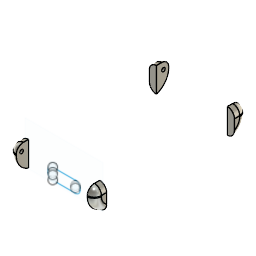
ILY Bracelet v2 v3 (Autodesk Fusion 360 design; units mm, degrees)
Autodesk Fusion 360 part; units mm, degrees
note: some values were not read from the file. Chosen so that the rebuilt part matches the saved one: which bodies a step acts on; which pieces of a blend or face edit are solid. Set by a fixed rule: which sketch regions a step uses.
sketch "Sketch1" plane through (0, 0, 0) normal (0, 0, 1) x (1, 0, 0)
  line L0 (0, 0) -> (22, 0)
  line L1 (22, 0) -> (22, 36)
  line L2 (22, 36) -> (0, 36)
  line L3 (0, 36) -> (0, 0)
  line L4 (1, 0.5) -> (21, 0.5)
  line L5 (21, 0.5) -> (21, 35)
  line L6 (21, 35) -> (1, 35)
  line L7 (1, 35) -> (1, 0.5)
  spline S0 degree 3 poles (15.3516, 13.4274) (15.5498, 13.4655) (15.7406, 13.3283) (15.7771, 13.115) knots 0 0 0 0 1 1 1 1
  spline S1 degree 3 poles (4.4385, 20.9712) (5.1653, 22.038) (6.0895, 22.8762) (7.1909, 23.4629) knots 0 0 0 0 1 1 1 1
  spline S2 degree 3 poles (10.9559, 18.0921) (10.1119, 18.0921) (9.4293, 17.4292) (9.4293, 16.6138) knots 0 0 0 0 1 1 1 1
  arc A0 (15.3516, 13.4274) -> (14.5896, 13.3512) centre (14.5065, 18.0307) cw
  spline S3 degree 3 poles (16.2692, 16.6049) (16.2692, 19.4777) (13.8838, 21.8094) (10.9482, 21.8094) knots 0 0 0 0 1 1 1 1
  spline S4 degree 3 poles (9.0696, 11.2849) (8.4311, 11.9491) (8.085, 12.3771) (7.5945, 13.2978) knots 0 0 0 0 1 1 1 1
  spline S5 degree 3 poles (14.4201, 22.7924) (12.3138, 23.9125) (9.6201, 23.9125) (7.5211, 22.7847) knots 0 0 0 0 1 1 1 1
  arc A1 (9.3264, 11.1706) -> (9.0696, 11.2849) centre (9.3232, 11.509) cw
  spline S6 degree 3 poles (13.2018, 11.7675) (13.4, 11.7142) (13.5101, 11.5008) (13.4587, 11.3027) knots 0 0 0 0 1 1 1 1
  spline S7 degree 3 poles (6.1556, 13.8541) (6.2292, 13.656) (6.1337, 13.435) (5.9428, 13.3664) knots 0 0 0 0 1 1 1 1
  arc A2 (17.51, 20.994) -> (17.4217, 20.4606) centre (17.1882, 20.7733) cw
  arc A3 (9.5982, 11.2874) -> (9.3264, 11.1706) centre (9.3177, 11.5655) cw
  arc A4 (6.3981, 24.5691) -> (6.5451, 25.0873) centre (6.7479, 24.7498) cw
  spline S8 degree 3 poles (10.9482, 21.8094) (8.8638, 21.8094) (6.9557, 20.6054) (6.0972, 18.7385) knots 0 0 0 0 1 1 1 1
  spline S9 degree 3 poles (12.7701, 11.1021) (11.7401, 11.4296) (11.0298, 11.8712) (10.2878, 12.6273) knots 0.072674 0.072674 0.072674 0.072674 1 1 1 1
  spline S10 degree 3 poles (14.7427, 14.3723) (13.4949, 14.3723) (12.4821, 15.3781) (12.4821, 16.6125) knots 0 0 0 0 1 1 1 1
  spline S11 degree 3 poles (10.9555, 18.8452) (12.203, 18.8452) (13.2161, 17.8394) (13.2161, 16.6049) knots 0 0 0 0 1 1 1 1
  spline S12 degree 3 poles (10.9797, 19.9501) (9.0937, 19.9501) (7.558, 18.449) (7.558, 16.6049) knots 0 0 0 0 1 1 1 1
  spline S13 degree 3 poles (6.0972, 18.7385) (5.8114, 18.1213) (5.6641, 17.3974) (5.6641, 16.6049) knots 0 0 0 0 1 1 1 1
  spline S14 degree 3 poles (5.4364, 19.0738) (6.4127, 21.2011) (8.5778, 22.579) (10.9482, 22.579) knots 0 0 0 0 1 1 1 1
  arc A5 (13.4587, 11.3027) -> (13.457, 11.2948) centre (13.104, 11.3734) cw
  arc A6 (5.4733, 13.5887) -> (4.9373, 16.6049) centre (13.7127, 16.6084) cw
  spline S15 degree 3 poles (10.9854, 25.4898) (9.5322, 25.4898) (8.1523, 25.1317) (6.8973, 24.4154) knots 0 0 0 0 1 1 1 1
  arc A7 (15.7771, 13.115) -> (15.4764, 12.673) centre (15.4052, 13.0447) cw
  arc A8 (12.7701, 11.1021) -> (13.457, 11.2948) centre (10.989, 18.773) ccw
  spline S16 degree 3 poles (7.5211, 22.7847) (6.5229, 22.2513) (5.6863, 21.4893) (5.0259, 20.5305) knots 0 0 0 0 1 1 1 1
  line L8 (14.589, 12.5816) -> (14.589, 12.5803)
  spline S17 degree 3 poles (10.8019, 13.1772) (11.5004, 12.4609) (12.1671, 12.0659) (13.2018, 11.7675) knots 0 0 0 0 1 1 1 1
  spline S18 degree 3 poles (8.2403, 13.6712) (8.7102, 12.7949) (9.034, 12.4215) (9.5982, 11.8272) knots 0 0 0 0 1 1 1 1
  spline S19 degree 3 poles (8.6953, 16.6049) (8.6953, 17.8394) (9.7081, 18.8452) (10.9555, 18.8452) knots 0 0 0 0 1 1 1 1
  spline S20 degree 3 poles (10.9854, 26.2518) (12.5484, 26.2518) (13.9137, 25.8937) (15.411, 25.0936) knots 0 0 0 0 1 1 1 1
  spline S21 degree 3 poles (7.5945, 13.2978) (7.0865, 14.2351) (6.8239, 15.3781) (6.8239, 16.6049) knots 0 0 0 0 1 1 1 1
  spline S22 degree 3 poles (13.2161, 16.6049) (13.2161, 15.7896) (13.8988, 15.1266) (14.7427, 15.1266) knots 0 0 0 0 1 1 1 1
  spline S23 degree 3 poles (10.9482, 22.579) (14.2877, 22.579) (17.0033, 19.9044) (17.0033, 16.6125) knots 0 0 0 0 1 1 1 1
  arc A9 (15.4764, 12.673) -> (14.589, 12.5816) centre (14.5393, 17.4162) cw
  arc A10 (6.5451, 25.0873) -> (10.9854, 26.2518) centre (10.9593, 17.3044) cw
  spline S24 degree 3 poles (14.589, 12.5803) (13.7156, 12.5803) (12.945, 12.8089) (12.3138, 13.2585) knots 0 0 0 0 1 1 1 1
  spline S25 degree 3 poles (6.8973, 24.4154) (6.7198, 24.3151) (6.501, 24.3849) (6.3981, 24.5691) knots 0 0 0 0 1 1 1 1
  spline S26 degree 3 poles (10.2878, 12.6273) (9.2601, 13.6865) (8.6953, 15.0962) (8.6953, 16.6049) knots 0 0 0 0 1 1 1 1
  arc A11 (4.5268, 20.4378) -> (4.4385, 20.9712) centre (4.759, 20.7502) cw
  arc A12 (15.411, 25.0936) -> (15.565, 24.5831) centre (15.2274, 24.7597) cw
  arc A13 (5.0259, 20.5305) -> (4.7395, 20.3692) centre (4.7494, 20.6866) cw
  spline S27 degree 3 poles (4.9373, 16.6049) (4.9373, 17.5193) (5.1062, 18.3512) (5.4364, 19.0738) knots 0 0 0 0 1 1 1 1
  spline S28 degree 3 poles (5.6641, 16.6049) (5.6641, 16.0106) (5.7152, 15.0733) (6.1556, 13.8541) knots 0 0 0 0 1 1 1 1
  spline S29 degree 3 poles (12.4821, 16.6125) (12.4824, 17.4279) (11.7998, 18.0921) (10.9559, 18.0921) knots 0 0 0 0 1 1 1 1
  arc A14 (10.5676, 16.6037) -> (11.3016, 16.6037) centre (10.9346, 16.6189) cw
  spline S30 degree 3 poles (14.3998, 16.6049) (14.3998, 18.449) (12.8656, 19.9501) (10.9797, 19.9501) knots 0 0 0 0 1 1 1 1
  spline S31 degree 3 poles (16.908, 20.5521) (16.2476, 21.5122) (15.411, 22.2666) (14.4201, 22.7924) knots 0 0 0 0 1 1 1 1
  spline S32 degree 3 poles (6.8239, 16.6049) (6.8239, 18.8681) (8.6879, 20.7121) (10.9781, 20.7121) knots 0 0 0 0 1 1 1 1
  spline S33 degree 3 poles (12.7253, 13.8909) (13.2463, 13.5252) (13.8556, 13.3512) (14.5896, 13.3512) knots 0 0 0 0 1 1 1 1
  spline S34 degree 3 poles (7.558, 16.6049) (7.558, 15.5076) (7.7926, 14.4942) (8.2403, 13.6712) knots 0 0 0 0 1 1 1 1
  spline S35 degree 3 poles (14.7427, 15.1266) (15.5866, 15.1266) (16.2692, 15.7896) (16.2692, 16.6049) knots 0 0 0 0 1 1 1 1
  spline S36 degree 3 poles (7.1909, 23.4629) (9.4954, 24.6961) (12.4459, 24.705) (14.7576, 23.4705) knots 0 0 0 0 1 1 1 1
  spline S37 degree 3 poles (9.4293, 16.6138) (9.4293, 15.3121) (9.9138, 14.0916) (10.8019, 13.1772) knots 0 0 0 0 1 1 1 1
  spline S38 degree 3 poles (15.0732, 24.4154) (13.6641, 25.1698) (12.4459, 25.4898) (10.9854, 25.4898) knots 0 0 0 0 1 1 1 1
  arc A15 (12.3138, 13.2585) -> (10.5676, 16.6037) centre (14.6665, 16.615) cw
  arc A16 (9.5982, 11.8272) -> (9.5982, 11.2874) centre (9.2999, 11.5573) cw
  arc A17 (12.7253, 13.8909) -> (11.3016, 16.6037) centre (14.6125, 16.6113) cw
  spline S39 degree 3 poles (17.0033, 16.6125) (17.0033, 15.3781) (15.9905, 14.3723) (14.7427, 14.3723) knots 0 0 0 0 1 1 1 1
  arc A18 (5.9428, 13.3664) -> (5.4733, 13.5887) centre (5.8147, 13.7029) cw
  arc A19 (4.7395, 20.3692) -> (4.5268, 20.4378) centre (4.7422, 20.7416) cw
  arc A20 (15.565, 24.5831) -> (15.2421, 24.3697) centre (15.237, 24.7284) cw
  spline S40 degree 3 poles (10.9781, 20.7121) (13.2682, 20.7121) (15.1335, 18.8681) (15.1335, 16.6049) knots 0 0 0 0 1 1 1 1
  arc A21 (15.1335, 16.6049) -> (14.3998, 16.6049) centre (14.7666, 16.5941) cw
  spline S41 degree 3 poles (14.7576, 23.4705) (15.8587, 22.8838) (16.7832, 22.0532) (17.51, 20.994) knots 0 0 0 0 1 1 1 1
  arc A22 (17.4217, 20.4606) -> (16.908, 20.5521) centre (17.2077, 20.747) cw
  arc A23 (15.2421, 24.3697) -> (15.0732, 24.4154) centre (15.2413, 24.7015) cw
  dimension "d1" = 22
  dimension "d2" = 36
  constraint horizontal L0
  constraint vertical L1
  constraint horizontal L2
  constraint vertical L3
  constraint coincident L0.start L3.end
  constraint horizontal L4
  constraint vertical L5
  constraint horizontal L6
  constraint vertical L7
  measures "d1" distance of L0.start L0.end
  measures "d2" distance of L0.start L2.end
extrude "Extrude1" add sketch "Sketch1" against normal blind 12 contours L0 L1 L2 L3 | L4 L5 L6 L7 | S0 A0 A7 A9 S24 A14 S33 A15 A17 | S1 S5 A2 S16 A11 A13 S31 S36 A19 S41 A22 | S2 S3 S6 S7 S8 S9 S10 S11 S13 S14 A5 A6 A8 S17 S19 S22 S23 S26 S27 S28 S29 S35 S37 S39 A18 | S4 A1 A3 S12 S18 S21 S30 S32 S34 A16 S40 A21 | A4 S15 S20 A10 S25 A12 S38 A20 A23 makes body 1
sketch "Sketch2" plane through (0, 0, 0) normal (0, -1, 0) x (1, 0, 0)
  line L0 (22, 0) -> (0, 0)
  line L1 (0, 0) -> (0, -12)
  line L2 (0, -12) -> (22, -12)
  line L3 (22, -12) -> (22, 0)
  arc A0 (6.505, -10.0575) -> (7.785, -11.34) centre (7.7875, -10.0575) ccw
  line L4 (6.505, -9.4575) -> (6.505, -10.0575)
  line L5 (7.785, -11.34) -> (14.17, -11.34)
  arc A1 (7.785, -8.175) -> (6.505, -9.4575) centre (7.785, -9.455) ccw
  line L6 (7.785, -8.175) -> (14.17, -8.175)
  arc A2 (15.45, -9.4575) -> (14.17, -8.175) centre (14.17, -9.455) ccw
  arc A3 (14.17, -11.34) -> (15.45, -10.0575) centre (14.1675, -10.0575) ccw
  line L7 (15.45, -9.4575) -> (15.45, -10.0575)
  constraint horizontal L6
  constraint vertical L7
  constraint tangent L6 A2
  constraint tangent A3 L7
extrude "Extrude2" cut sketch "Sketch1" against normal blind 11.5 contours L4 L5 L6 L7 | S0 A0 A7 A9 S24 A14 S33 A15 A17 | S1 S5 A2 S16 A11 A13 S31 S36 A19 S41 A22 | S2 S3 S6 S7 S8 S9 S10 S11 S13 S14 A5 A6 A8 S17 S19 S22 S23 S26 S27 S28 S29 S35 S37 S39 A18 | S4 A1 A3 S12 S18 S21 S30 S32 S34 A16 S40 A21 | A4 S15 S20 A10 S25 A12 S38 A20 A23 bodies 1
extrude "Extrude3" cut sketch "Sketch2" against normal blind 5 contours A0 L4 L5 A1 L6 A2 A3 L7 bodies 1
extrude "Extrude4" add sketch "Sketch1" against normal blind 0.5 contours L4 L5 L6 L7 | S0 A0 A7 A9 S24 A14 S33 A15 A17 | S1 S5 A2 S16 A11 A13 S31 S36 A19 S41 A22 | S2 S3 S6 S7 S8 S9 S10 S11 S13 S14 A5 A6 A8 S17 S19 S22 S23 S26 S27 S28 S29 S35 S37 S39 A18 | S4 A1 A3 S12 S18 S21 S30 S32 S34 A16 S40 A21 | A4 S15 S20 A10 S25 A12 S38 A20 A23 bodies 1
extrude "Extrude5" cut sketch "Sketch1" against normal blind 0.25 contours S0 A0 A7 A9 S24 A14 S33 A15 A17 | S1 S5 A2 S16 A11 A13 S31 S36 A19 S41 A22 | S2 S3 S6 S7 S8 S9 S10 S11 S13 S14 A5 A6 A8 S17 S19 S22 S23 S26 S27 S28 S29 S35 S37 S39 A18 | S4 A1 A3 S12 S18 S21 S30 S32 S34 A16 S40 A21 | A4 S15 S20 A10 S25 A12 S38 A20 A23 bodies 1
chamfer "Chamfer1" distance 7 distance2 0.7 1 edges at (22, 0, -6) measured on face at (22, 12, -4) on bodies 1
fillet "Fillet1" radius 1 2 edges at (21.3, 0, -6) (22, 7, -6) on bodies 1
chamfer "Chamfer2" distance 0.75 distance2 7 1 edges at (22, 36, -6) measured on face at (14.6667, 36, -8) on bodies 1
chamfer "Chamfer3" distance 7 distance2 0.7 1 edges at (0, 36, -6) measured on face at (0, 24, -4) on bodies 1
chamfer "Chamfer4" distance 0.7 distance2 7 1 edges at (0, 0, -6) measured on face at (9.3933, 0, -2.725) on bodies 1
fillet "Fillet2" radius 1 6 edges at (0.7, 0, -6) (0, 7, -6) (21.25, 36, -6) (22, 29, -6) (0.7, 36, -6) (0, 29, -6) on bodies 1
sketch "Sketch3" plane through (0, 0, 0) normal (0, -1, 0) x (1, 0, 0)
  line L0 (1.605, 0) -> (1.605, -12)
  line L1 (1.605, -12) -> (20.395, -12)
  line L2 (20.395, -12) -> (20.395, 0)
  line L3 (20.395, 0) -> (1.605, 0)
  line L4 (6.505, -10.0575) -> (6.505, -9.4575)
  arc A0 (7.785, -8.175) -> (6.505, -9.4575) centre (7.785, -9.455) ccw
  line L5 (7.785, -8.175) -> (14.17, -8.175)
  arc A1 (15.45, -9.4575) -> (14.17, -8.175) centre (14.17, -9.455) ccw
  line L6 (15.45, -9.4575) -> (15.45, -10.0575)
  arc A2 (14.17, -11.34) -> (15.45, -10.0575) centre (14.1675, -10.0575) ccw
  line L7 (14.17, -11.34) -> (7.785, -11.34)
  arc A3 (6.505, -10.0575) -> (7.785, -11.34) centre (7.7875, -10.0575) ccw
  line L8 (21, -4.75) -> (21, -8)
  line L9 (1, -8) -> (1, -4.75)
  line L10 (1, -4.75) -> (0, -4.75)
  line L11 (21, -4.75) -> (22, -4.75)
  line L12 (22, -4.75) -> (23, -4.75)
  line L13 (23, -4.75) -> (23, -12)
  line L14 (23, -12) -> (22, -12)
  line L15 (0, -4.75) -> (-1, -4.75)
  line L16 (-1, -4.75) -> (-1, -12)
  line L17 (-1, -12) -> (0, -12)
  line L18 (21, -8) -> (21, -12)
  line L19 (21, -12) -> (22, -12)
  line L20 (1, -8) -> (1, -12)
  line L21 (1, -12) -> (0, -12)
  constraint vertical L8
  constraint vertical L9
  constraint horizontal L10
  constraint horizontal L11
  constraint horizontal L12
  constraint vertical L13
  constraint horizontal L14
  constraint horizontal L15
  constraint vertical L16
  constraint horizontal L17
  constraint parallel L8 L18
  constraint perpendicular L18 L19
  constraint perpendicular L1 L20
extrude "Extrude6" add sketch "Sketch3" against normal blind 11 separate body contours L8 L11 L12 L13 L14 L18 L19 | L9 L10 L15 L16 L17 L20 L21 makes body 2 at (23, 3.6667, -7.1667) makes body 3 at (-1, 3.6667, -7.1667)
extrude "Extrude7" add 2 faces at (21.6667, 0, -7.1667) (0, 0, -7.1667) along direction (0, -1, 0) blind 3.5 on bodies 2 3 bodies 2 3
fillet "Fillet3" radius 5 3 edges at (22, -3.5, -12) (-0.5, -3.5, -12) (0.5, -3.5, -12) on bodies 2 3
fillet "Fillet4" radius 2 2 edges at (22, -3.5, -4.75) (0, -3.5, -4.75) on bodies 2 3
fillet "Fillet5" radius 2 10 edges at (23, 6.25, -12) (23, -2.0355, -10.5355) (23, -3.5, -6.875) (23, -2.9142, -5.3358) (23, 4.75, -4.75) (-1, 6.25, -12) (-1, -2.0355, -10.5355) (-1, -3.5, -6.875) (-1, -2.9142, -5.3358) (-1, 4.75, -4.75) on bodies 2 3
chamfer "Chamfer5" distance 2 distance2 5 6 edges at (23, 11, -8.375) (22.4142, 11, -11.4142) (22.4142, 11, -5.3358) (-1, 11, -8.375) (-0.4142, 11, -5.3358) (-0.4142, 11, -11.4142) measured on face at (21.6667, 11, -7.8333) measured on face at (22.9909, 7.8333, -10.1901) measured on face at (22.9977, 6.8333, -6.6548) measured on face at (0.3333, 11, -7.8332) measured on face at (0.9045, 6.8333, -4.7523) measured on face at (-0.2829, 4.666, -11.5345) on bodies 2 3
mirror "Mirror1" about plane through (0, 0, 0) normal (0, 1, 0) of bodies 2 3 makes body 4 at (21, -2, -7.1667) makes body 5 at (1, -2.0017, -7.1667)
sketch "Sketch4" plane through (21, 0, 0) normal (-1, 0, 0) x (0, -1, 0)
  line L0 (-11, -10) -> (-6, -12)
  line L1 (-6, -12) -> (-1.5, -12)
  arc A0 (-1.5, -12) -> (3.5, -7) centre (-1.5, -7) ccw
  line L2 (3.5, -7) -> (3.5, -6.75)
  arc A1 (3.5, -6.75) -> (1.5, -4.75) centre (1.5, -6.75) ccw
  line L3 (1.5, -4.75) -> (-6, -4.75)
  line L4 (-6, -4.75) -> (-11, -6.75)
  line L5 (-11, -6.75) -> (-11, -10)
  circle A2 centre (2, -6.75) radius 0.5
  dimension "d42" = 1
  measures "d42" diameter of A2
move_body "Move1" bodies 4 5 to x (1, 0, 0) y (0, 1, 0) z (0, 0, 1) at (0, 36, 0)
extrude "Extrude8" cut sketch "Sketch4" against normal blind 1 contours A2 bodies 2
sketch "Sketch5" plane through (1, 0, 0) normal (1, 0, 0) x (0, 1, 0)
  line L0 (11, -6.75) -> (6, -4.75)
  line L1 (6, -4.75) -> (-1.5, -4.75)
  arc A0 (-1.5, -4.75) -> (-3.5, -6.75) centre (-1.5, -6.75) ccw
  line L2 (-3.5, -6.75) -> (-3.5, -7)
  arc A1 (-3.5, -7) -> (1.5, -12) centre (1.5, -7) ccw
  line L3 (1.5, -12) -> (6, -12)
  line L4 (6, -12) -> (11, -10)
  line L5 (11, -10) -> (11, -6.75)
  circle A2 centre (-2, -6.75) radius 0.5
  dimension "d46" = 1
  measures "d46" diameter of A2
extrude "Extrude9" cut sketch "Sketch5" against normal blind 1 contours A2 bodies 3
delete_body "RemoveBody1" bodies 4
delete_body "RemoveBody2" bodies 5
mirror "Mirror2" about plane through (0, 0, 0) normal (0, 1, 0) of bodies 2 3 makes body 6 at (21, -1.9981, -7.8582) makes body 7 at (1, -1.9998, -7.8582)
move_body "Move2" bodies 6 7 to x (1, 0, 0) y (0, 1, 0) z (0, 0, 1) at (0, 36, 0)
fillet "Fillet6" radius 1 16 edges at (21.9986, 28.9999, 0) (21.67, 32.0798, 0) (21.0198, 35.7438, 0) (10.9782, 36, 0) (0.934, 35.7415, 0) (0.3075, 32.0746, 0) (0.0012, 28.9999, 0) (0, 18, 0) (0.0012, 7.0001, 0) (0.3075, 3.9254, 0) (0.934, 0.2585, 0) (11, 0, 0) (21.066, 0.2585, 0) (21.6925, 3.9254, 0) (21.9988, 7.0001, 0) (22, 17.9982, 0) on bodies 1
sketch "Sketch7" plane through (0, 0, 0) normal (0, 1, 0) x (1, 0, 0)
  line L0 (-1, 4.5) -> (0.6, 4.5)
  line L1 (1, 9.5) -> (21, 9.5)
  line L2 (21.4, 4.5) -> (23.7846, 4.5)
  line L3 (21.4, 9.5) -> (21, 9.5)
  line L4 (1, 9.5) -> (0.6, 9.5)
  arc A0 (21.4, 8.625) -> (21.4, 9.375) centre (21.4, 9) ccw
  line L5 (21.4, 4.5) -> (21.4, 8.625)
  line L6 (21.4, 9.375) -> (21.4, 9.5)
  arc A1 (0.6, 9.375) -> (0.6, 8.625) centre (0.6, 9) ccw
  line L7 (0.6, 9.5) -> (0.6, 9.375)
  line L8 (0.6, 8.625) -> (0.6, 4.5)
  dimension "d55" = 0.75
  dimension "d56" = 0.75
  constraint horizontal L0
  constraint perpendicular L1 L5
  constraint parallel L1 L4
  constraint perpendicular L0 L7
  constraint coincident A1.centre L7
  constraint coincident A0.end L5
  constraint collinear L5 L6
  constraint collinear L7 L8
  measures "d55" diameter of A1
  measures "d56" diameter of A0
sketch "Sketch8" plane through (0, 0, 0) normal (1, 0, 0) x (0, 1, 0)
  line L0 (36, 0) -> (36, -12)
  line L1 (0, -12) -> (0, 0)
  constraint vertical L0
  constraint vertical L1
  constraint coincident L1.end origin
split "Split5" by curves path "Sketch8" along L1 L0 bodies 7 6 3 2 makes body 8 at (21, 2.5, -7.1667) makes body 9 at (1, 2.5017, -7.1667) makes body 10 at (21, 33.5, -7.1667) makes body 11 at (1, 33.4983, -7.1667)
combine "Combine2" [rolled back]
split "Split6" [rolled back]
combine "Combine3" [rolled back]
move_body "Move3" [rolled back]
move_body "Move4" [rolled back]
split "Split4" [suppressed]
split "Split3" [suppressed]
split "Split2" [suppressed]
combine "Combine1" [suppressed]
split "Split1" [suppressed]
hidden bodies 8 10 11 9 1
